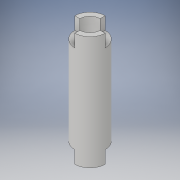
# Autodesk Inventor part: Steckhülse
Saved by Autodesk Inventor 2017 (Build 210142000, 142)
## iProperties
Part Number: Steckhülse
Material: Generisch
Document SubType Name: Modeling
Designer: Benjamin
Density: 1 g/cm^3
Appearance: Vorgabe
Author: Benjamin
Autodesk Inventor part; units mm, degrees
ref_plane "YZ Plane" through (0, 0, 0) normal (1, 0, 0) x (0, 1, 0)
ref_plane "XZ Plane" through (0, 0, 0) normal (0, 1, 0) x (-1, 0, 0)
ref_plane "XY Plane" through (0, 0, 0) normal (0, 0, 1) x (1, 0, 0)
sketch "Skizze1" plane through (0, 0, 0) normal (0, 0, 1) x (1, 0, 0)
  circle A0 centre (0, 0) radius 6
  dimension "d0" = 12
  constraints: 1 centre point, 1 coincident
  measures "d0" diameter of A0
extrude "Extrusion1" add sketch "Skizze1" along normal blind 35
sketch "Skizze2" plane through (0, 0, 0) normal (0, 0, -1) x (-1, 0, 0)
  circle A0 centre (0, 0) radius 4
  dimension "d3" = 8
  constraints: 1 centre point, 1 coincident
  measures "d3" diameter of A0
extrude "Extrusion2" cut sketch "Skizze2" against normal blind 35
sketch "Skizze9" plane through (0, 0, 35) normal (0, 0, 1) x (1, 0, 0)
  arc A0 (0, 6) -> (-6, 0) centre (0, 0) ccw
  arc A1 (0, 4) -> (-4, 0) centre (0, 0) ccw
  line L0 (0, 4) -> (0, 6)
  line L1 (4, 0) -> (6, 0)
  line L2 (-4, 0) -> (-6, 0)
  arc A2 (0, -6) -> (6, 0) centre (0, 0) ccw
  arc A3 (0, -4) -> (4, 0) centre (0, 0) ccw
  line L3 (0, -4) -> (0, -6)
  constraints: 9 point on circle, 8 end point, 4 centre point, 2 coincident, 2 horizontal, 2 vertical
sketch "Skizze9 outline for Extrusion8" plane through (0, 0, 35) normal (0, 0, 1) x (1, 0, 0)
  line L0 (0, 6) -> (0, 4)
  arc A0 (0, 4) -> (-4, 0) centre (0, 0) ccw
  line L1 (-4, 0) -> (-6, 0)
  arc A1 (-6, 0) -> (0, 6) centre (0, 0) cw
  line L2 (4, 0) -> (6, 0)
  arc A2 (6, 0) -> (0, -6) centre (0, 0) cw
  line L3 (0, -6) -> (0, -4)
  arc A3 (0, -4) -> (4, 0) centre (0, 0) ccw
extrude "Extrusion8" add sketch "Skizze9 outline for Extrusion8" along normal blind 5
sketch "Skizze10" plane through (0, 0, 0) normal (0, 0, -1) x (-1, 0, 0)
  line L0 (0, -4) -> (0, -6) projected
  line L1 (-4, 0) -> (-6, 0) projected
  line L2 (-6, 0) -> (-4, 0)
  line L3 (0, 6) -> (0, 4) projected
  line L4 (0, -4) -> (0, -6)
  line L5 (-4, 0) -> (-6, 0)
  arc A0 (-6, 0) -> (0, -6) centre (0, 0) ccw
  arc A1 (6, 0) -> (0, 6) centre (0, 0) ccw
  arc A2 (4, 0) -> (0, 4) centre (0, 0) ccw
  line L6 (4, 0) -> (6, 0) projected
  line L7 (6, 0) -> (4, 0)
  arc A3 (-4, 0) -> (0, -4) centre (0, 0) ccw
  constraints: 9 end point, 8 point on circle, 4 centre point, 2 collinear, 1 coincident, 1 horizontal, 1 vertical
extrude "Extrusion9" add sketch "Skizze10" along normal blind 5
